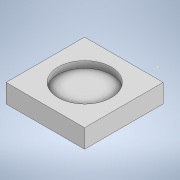
# Autodesk Inventor part: LED
Saved by Autodesk Inventor 2021 (Build 250183000, 183)
## iProperties
Created: 2021-03-11
Part Number: LED
Material: Generic
Document SubType Name: Modeling
Designer: bddamman
Density: 1 g/cm^3
Appearance: Default
Author: bddamman
Autodesk Inventor part; units mm, degrees
ref_plane "YZ Plane" through (0, 0, 0) normal (1, 0, 0) x (0, 1, 0)
ref_plane "XZ Plane" through (0, 0, 0) normal (0, 1, 0) x (-1, 0, 0)
ref_plane "XY Plane" through (0, 0, 0) normal (0, 0, 1) x (1, 0, 0)
sketch "Sketch1" plane through (0, 0, 0) normal (0, 1, 0) x (-1, 0, 0)
  line L0 (2.3791, 3.4135) -> (-0.6209, 3.4135)
  line L1 (-0.6209, 3.4135) -> (-0.6209, 0.4135)
  line L2 (-0.6209, 0.4135) -> (2.3791, 0.4135)
  line L3 (2.3791, 0.4135) -> (2.3791, 3.4135)
  point P0 (0, 0)
  dimension "d0" = 3
  dimension "d1" = 3
  constraints: 8 end point, 2 parallel, 1 horizontal, 1 perpendicular
  measures "d0" distance of L2.end L1.end
  measures "d1" distance of L1.end L0.end
extrude "Extrusion1" add sketch "Sketch1" along normal blind 0.7112
sketch "Sketch2" plane through (0, 0.7112, 0) normal (0, 1, 0) x (1, 0, 0)
  point P0 (0, 0)
sketch "Sketch3" plane through (0, 0.7112, 0) normal (0, 1, 0) x (1, 0, 0)
  point P0 (0, 0)
  point P1 (-0.8772, -1.9095)
hole "Hole1" at (-0.8772, 0.7112, 1.9095) direction (0, -1, 0) diameter 2.032 depth 0.254
body "Solid1"
